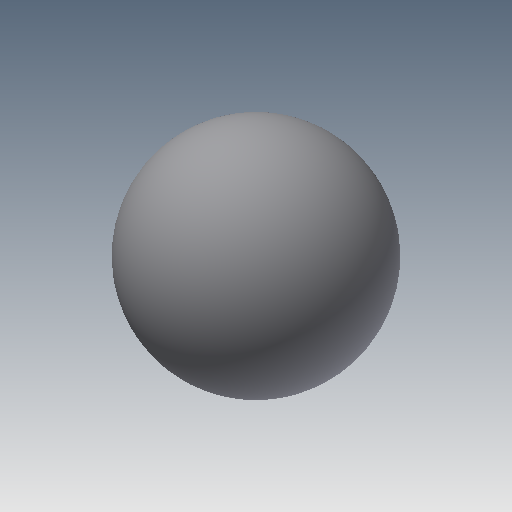
# Autodesk Inventor part: A-2015_ball
Saved by Autodesk Inventor 2019.4 (Build 234330000, 330)
## iProperties
Category: PARTsolutions
Company: NMB
Created: 2019-11-12
Part Number: A-2015_ball
Material: 一般
Catalog Web Link: www.cadenas.de
Description: Radial Ball Bearings (A series)  OT ball-Radial Ball Bearings (A series)  Open Type
Vendor: NMB
Document SubType Name: Modeling
Designer: psadmin
Manufacturer: NMB
Mass: 0.00209479 g
Surface Area: 0.079173 cm^2
Volume: 0.00209479 cm^3
Density: 1 g/cm^3
Appearance: PSOLRGB-192-192-192
PSOL_IDENT_0: {$CADENAS_DATA\23d-libs\nmb\pbbp\radial_ball_bear_thin_secti\rbb_as\as_open_ball.prj},197 {VTYP=3D},
PSOL_IDENT_1: {NB=A-2015_ball},{LINA=A-2015_ball},{NN=Radial Ball Bearings (A series)  OT ball},{DATE=11.11.2013 0
PSOL_IDENT_2: 5:13:38},{GEOMDATE=29.10.2013 14:02:00},{VERSION=},{LINEID=870},{WBVAR=},{WBNUMERIC=}  {NB=A-2015_ba
PSOL_IDENT_3: ll},{LINA=A-2015_ball},{KT=DUMMY},{IDNR=},{PN=A-2015},{SHLD=open},{FLANG=unflanged},{SD=15.000},{D=2
PSOL_IDENT_4: 0.000},{B=3.500},{SR=0.15},{BCZ=14},{DW=1.5875},{LI=16.40},{LO=18.43},{D1=0.000},{C1=0.00},{D2=0.0},
PSOL_IDENT_5: {C2=0.00},{COR=582},{CR=1085},{PCD=17.500},{U=19.088},{W=15.913},{Y=0.794},{Z=0.794},{AA=0.000},{AC=
PSOL_IDENT_6: 0.00},{AD=0.000},{AF=0.00},{AQ=0.00},{AH=0.00},{AI=0.00},{AJ=0.00}
NN: Radial Ball Bearings (A series)  OT ball
NT: Radial Ball Bearings (A series)  Open Type
NB: A-2015_ball
NBSYN: $PN._ball
LINA: A-2015_ball
PN: A-2015
SHLD: open
FLANG: unflanged
SD: 15
D: 20
B: 3.5
SR: 0.15
BCZ: 14
DW: 1.5875
LI: 16.4
LO: 18.43
D1: 0
C1: 0
D2: 0
C2: 0
COR: 582
CR: 1085
PCD: 17.5
U: 19.088
W: 15.913
Y: 0.794
Z: 0.794
AA: 0
AC: 0
AD: 0
AF: 0
AQ: 0
AH: 0
AI: 0
AJ: 0
SUPPLIER: NMB
ARTICLENO: A-2015_ball
BOMINFO: A-2015_ball
CREATOR: CADENAS GmbH
Title: A-2015_ball
Author: Cadenas PARTsolutions
Comments: Radial Ball Bearings (A series)  Open Type
Autodesk Inventor part; units mm, degrees
sketch "Sketch_1" plane through (0, 0, 0) normal (0, 0, 1) x (1, 0, 0)
  line L0 (0.7937, 0) -> (-0.7937, 0)
  arc A0 (0.7937, 0) -> (-0.7937, 0) centre (0, 0) ccw
  line L1 (0.7937, 0) -> (-0.7937, 0)
  constraints: 4 end point, 2 point on circle, 1 centre point
revolve "Revolution1" add sketch "Sketch_1" angle 360 about axis through (0.7937, 0, 0) along (1, 0, 0)
ref_plane "1_XY" through (0, 0, 0) normal (0, 0, 1) x (1, 0, 0)
ref_plane "1_YZ" through (0, 0, 0) normal (1, 0, 0) x (0, 1, 0)
ref_plane "1_ZX" through (0, 0, 0) normal (0, 1, 0) x (0, 0, 1)
body "Solid1"
